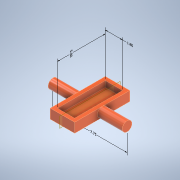
# Autodesk Inventor part: connectorToTubeBrackets
Saved by Autodesk Inventor 2021 (Build 250183000, 183)
## iProperties
Created: 2020-07-21
Part Number: connectorToTubeBrackets
Material: PC/ABS Plastic
Document SubType Name: Modeling
Designer: robst
Density: 0.357273 g/cm^3
Appearance: Smooth - Light Orange
Author: robst
Autodesk Inventor part; units mm, degrees
ref_plane "XZ Plane" through (0, 0, 0) normal (0, 1, 0) x (-1, 0, 0)
ref_plane "XY Plane" through (0, 0, 0) normal (0, 0, 1) x (1, 0, 0)
sketch "Sketch1" plane through (0, 0, 0) normal (0, 1, 0) x (-1, 0, 0)
  line L0 (32.385, 73.025) -> (-32.385, 73.025)
  line L1 (-32.385, 73.025) -> (-32.385, -73.025)
  line L2 (-32.385, -73.025) -> (32.385, -73.025)
  line L3 (32.385, -73.025) -> (32.385, 73.025)
  line L4 (32.385, 73.025) -> (-32.385, -73.025) construction
  line L5 (-32.385, 73.025) -> (32.385, -73.025) construction
  point P0 (0, 0)
  dimension "outerWidth" = 64.77
  dimension "outerLength" = 146.05
  constraints: 12 end point, 2 midpoint, 2 parallel, 1 horizontal, 1 perpendicular
  measures "outerWidth" distance of L1.end L2.end
  measures "outerLength" distance of L2.end L0.start
extrude "Extrusion1" add sketch "Sketch1" against normal blind 9.525
sketch "Sketch2" plane through (0, 0, 0) normal (0, 1, 0) x (1, 0, 0)
  line L0 (32.385, -73.025) -> (32.385, 73.025)
  line L1 (32.385, 73.025) -> (-32.385, 73.025)
  line L2 (-32.385, 73.025) -> (-32.385, -73.025)
  line L3 (-32.385, -73.025) -> (32.385, -73.025)
  line L4 (32.385, -73.025) -> (-32.385, 73.025) construction
  line L5 (32.385, 73.025) -> (-32.385, -73.025) construction
  line L6 (22.86, -63.5) -> (22.86, 63.5)
  line L7 (22.86, 63.5) -> (-22.86, 63.5)
  line L8 (-22.86, 63.5) -> (-22.86, -63.5)
  line L9 (-22.86, -63.5) -> (22.86, -63.5)
  line L10 (22.86, -63.5) -> (-22.86, 63.5) construction
  line L11 (22.86, 63.5) -> (-22.86, -63.5) construction
  line L12 (32.385, 73.025) -> (-32.385, 73.025) projected
  line L13 (-32.385, 73.025) -> (-32.385, -73.025) projected
  point P0 (0, 0)
  dimension "wallThickness" = 9.525
  dimension "d5" = 9.525
  constraints: 24 end point, 4 midpoint, 4 parallel, 2 collinear, 2 perpendicular, 1 vertical
  measures "wallThickness" distance between parallel lines of L7 L1
  measures "d5" distance between parallel lines of L2 L8
extrude "Extrusion2" add sketch "Sketch2" along normal blind 15.875
sketch "Sketch3" plane through (32.385, -9.525, 73.025) normal (1, 0, 0) x (0, 0, -1)
  circle A0 centre (73.025, 12.7) radius 12.7
  line L0 (0, 25.4) -> (146.05, 25.4) projected
  line L1 (0, 25.4) -> (0, 0) projected
  point P0 (73.025, 9.525)
  dimension "postDiameter" = 25.4
  dimension "d15" = 12.7
  dimension "d19" = 73.025
  constraints: 1 centre point
  measures "postDiameter" diameter of A0
  measures "d15" distance from line of A0.centre L0
  measures "d19" distance from line of A0.centre L1
extrude "Extrusion3" add sketch "Sketch3" along normal blind 66.04
mirror "Mirror1" about plane through (0, 0, 0) normal (1, 0, 0) of "Extrusion3"
equation "\"outerWidth\" = innerWidth + 2 * wallThickness"
equation "\"outerLength\" = innerLength + 2 * wallThickness"
equation "\"d2\" = wallThickness"
equation "\"d5\" = wallThickness"
equation "\"height\" = outerHeight - wallThickness"
equation "\"d15\" = 0.5 * outerHeight"
equation "\"d19\" = 0.5 * outerLength"
equation "\"d16\" = -0.5 * outerWidth + 0.5 * width"
equation "\"innerWidth\" = 45.72"
equation "\"innerLength\" = 127"
equation "\"width\" = 196.85"
equation "\"outerHeight\" = 25.4"
body "Solid1"
